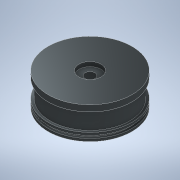
# Autodesk Inventor part: Верхняя часть поршня
Saved by Autodesk Inventor 2021 (Build 250183000, 183)
## iProperties
Created: 2020-10-24
Part Number: Верхняя часть поршня
Material: Чугун, серый
Document SubType Name: Modeling
Designer: Тимоха
Density: 7.15 g/cm^3
Appearance: Чугун серый
Mass: 61164.2 g
Surface Area: 6102.27 cm^2
Volume: 8554.43 cm^3
Author: Тимоха
Autodesk Inventor part; units mm, degrees
ref_plane "YZ Plane" through (0, 0, 0) normal (1, 0, 0) x (0, 1, 0)
ref_plane "XZ Plane" through (0, 0, 0) normal (0, 1, 0) x (-1, 0, 0)
ref_plane "XY Plane" through (0, 0, 0) normal (0, 0, 1) x (1, 0, 0)
sketch "Эскиз1" plane through (0, 0, 0) normal (0, 0, 1) x (1, 0, 0)
  line L0 (49.9998, 0) -> (189, 0)
  line L1 (189, 0) -> (189, -28)
  line L2 (189, -28) -> (178, -28)
  line L3 (178, -28) -> (178, -108)
  line L4 (178, -108) -> (189, -108)
  line L5 (149, -106) -> (152.99, -60.3945)
  line L6 (137.0508, -43) -> (70.9998, -43)
  line L7 (54.9998, -59) -> (54.9998, -152)
  line L8 (27.4998, -84) -> (22.4998, -84)
  line L9 (22.4998, -84) -> (22.4998, -20)
  line L10 (22.4998, -20) -> (49.9998, -20)
  line L11 (49.9998, -20) -> (49.9998, 0)
  arc A0 (70.9998, -43) -> (54.9998, -59) centre (70.9998, -59) ccw
  arc A1 (152.99, -60.3945) -> (137.0508, -43) centre (137.0508, -59) ccw
  arc A2 (37.4998, -94) -> (27.4998, -84) centre (27.4998, -94) ccw
  line L12 (0, 0) -> (0, 25.6698)
  line L13 (189, -108) -> (189, -120)
  line L14 (189, -144) -> (169, -144)
  line L15 (169, -144) -> (169, -152)
  line L16 (189, -144) -> (189, -132)
  line L17 (189, -132) -> (178, -132)
  line L18 (178, -132) -> (178, -120)
  line L19 (178, -120) -> (189, -120)
  line L20 (189, -108) -> (189, -120)
  line L21 (149, -152) -> (149, -106)
  line L22 (37.4998, -140) -> (37.4998, -94)
  line L23 (169, -152) -> (149, -152)
  line L24 (54.9998, -152) -> (39.9998, -152)
  line L25 (39.9998, -152) -> (39.9998, -140)
  line L26 (39.9998, -140) -> (37.4998, -140)
  point P0 (154.5118, -43)
  point P1 (54.9998, -43)
  point P2 (37.4998, -84)
  dimension "d0" = 189
  dimension "d1" = 28
  dimension "d2" = 11
  dimension "d3" = 80
  dimension "d10" = 63
  dimension "d11" = 99.512
  dimension "d16" = 15
  dimension "d17" = 64
  dimension "d18" = 27.5
  dimension "d24" = 16
  dimension "d25" = 16
  dimension "d26" = 10
  dimension "d29" = 20
  dimension "d30" = 8
  dimension "d31" = 12
  dimension "d32" = 11
  dimension "d33" = 12
  dimension "d34" = 12
  dimension "d35" = 46
  dimension "d36" = 93
  dimension "d37" = 46
  dimension "d38" = 15
  dimension "d39" = 20
  constraints: 54 end point, 14 perpendicular, 6 point on circle, 6 point on line, 5 tangent, 5 vertical, 4 horizontal, 3 centre point, 1 collinear
  measures "d0" distance of L12.start L0.end
  measures "d1" distance of L0.end L1.end
  measures "d2" distance of L1.end L2.end
  measures "d3" distance of L2.end L3.end
  measures "d10" vertical distance of L5.start point (154.512, -43)
  measures "d11" distance of point (154.512, -43) point (55, -43)
  measures "d16" distance of point (37.5, -84) L8.end
  measures "d17" distance of L8.end L9.end
  measures "d18" distance of L9.end L10.end
  measures "d24" radius of A0
  measures "d25" radius of A1
  measures "d26" radius of A2
  measures "d29" distance of L14.start L14.end
  measures "d30" distance of L14.end L15.end
  measures "d31" distance of L16.end L14.start
  measures "d32" distance of L16.end L17.end
  measures "d33" distance of L17.end L18.end
  measures "d34" distance of L4.end L13.end
  measures "d35" distance of L21.start L5.start
  measures "d36" distance of L7.start L7.end
  measures "d37" distance of L22.start L22.end
  measures "d38" distance of L7.end L24.end
  measures "d39" distance of L10.end L0.start
revolve "Вращение1" add sketch "Эскиз1" angle 360 about axis through (0, 0, 0) along (0, 1, 0)
